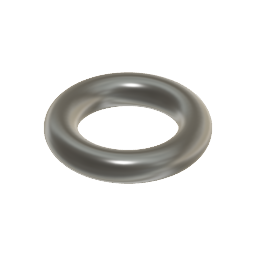
torusplayerpiece2 (Autodesk Fusion 360 archive; units mm, degrees)
design "torus2"
Autodesk Fusion 360 part; units mm, degrees
sketch "Sketch1" plane through (0, 0, 0) normal (0, 0, 1) x (1, 0, 0)
torus "TorusPrimitive1" add centre line diameter 22.86 section diameter 5.7912 placed x (1, 0, 0) y (0, 1, 0) z (0, 0, 1) at (0, 0, 0)

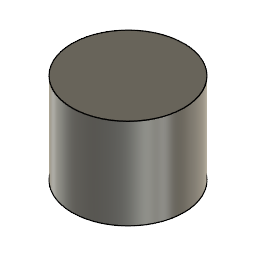
design "playerbase2"
Autodesk Fusion 360 part; units mm, degrees
sketch "Sketch1" plane through (0, 0, 0) normal (0, 0, 1) x (1, 0, 0)
  circle A0 centre (0, 0) radius 2.3495
  dimension "d1" = 4.699
  constraint coincident A0.centre origin
  measures "d1" diameter of A0
extrude "Extrude1" add sketch "Sketch1" along normal blind 3.81
